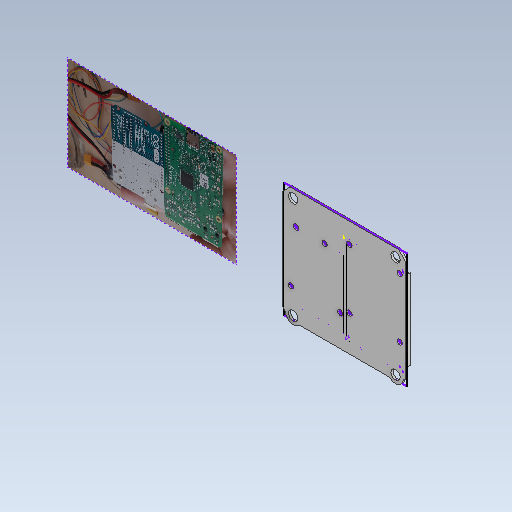
# Autodesk Inventor part: Крепление плат
Saved by Autodesk Inventor 2020 (Build 240168000, 168)
## iProperties
Created: 2021-04-20
Part Number: Крепление плат
Material: Типовые
Document SubType Name: Modeling
Designer: I_Love_U_Bogdan
Density: 1 g/cm^3
Appearance: По умолчанию
Author: I_Love_U_Bogdan
Autodesk Inventor part; units mm, degrees
ref_plane "YZ Plane" through (0, 0, 0) normal (1, 0, 0) x (0, 1, 0)
ref_plane "XZ Plane" through (0, 0, 0) normal (0, 1, 0) x (-1, 0, 0)
ref_plane "XY Plane" through (0, 0, 0) normal (0, 0, 1) x (1, 0, 0)
sketch "Эскиз2" plane through (0, 0, 0) normal (0, 0, 1) x (1, 0, 0)
  line L0 (-106.4716, 15.9838) -> (-106.4716, -76.8287) construction
  line L1 (-106.4716, -76.8287) -> (-271.4716, -76.8287) construction
  line L2 (-271.4716, -76.8287) -> (-271.4716, 15.9838) construction
  line L3 (-271.4716, 15.9838) -> (-106.4716, 15.9838) construction
  line L4 (4.5, 0) -> (54.5, 0)
  line L5 (57.5, -3) -> (57.5, -82)
  line L6 (54.5, -85) -> (4.5, -85)
  line L7 (1.5, -82) -> (1.5, -3)
  circle A0 centre (5, -3.5) radius 1.5
  circle A1 centre (54, -3.5) radius 1.5
  circle A2 centre (5, -61.5) radius 1.5
  circle A3 centre (54, -61.5) radius 1.5
  line L8 (-54.8, -14.8714) -> (-54.8, -80.9714)
  line L9 (-54.8, -80.9714) -> (-1.5, -80.9714)
  line L10 (-1.5, -80.9714) -> (-1.5, -14.8714)
  line L11 (-49.8, -11.8527) -> (-48.1279, -11.8527) construction
  circle A4 centre (-47.2, -14.8714) radius 1.5
  circle A5 centre (-19.3, -14.8714) radius 1.5
  circle A6 centre (-4.1, -65.6714) radius 1.5
  circle A7 centre (-52.3, -66.9714) radius 1.5
  line L12 (-16.4799, -14.8714) -> (-1.5, -14.8714)
  line L13 (-54.8, -14.8714) -> (-52.8, -14.8714)
  arc A8 (4.5, 0) -> (1.5, -3) centre (4.5, -3) ccw
  arc A9 (57.5, -3) -> (54.5, 0) centre (54.5, -3) ccw
  arc A10 (54.5, -85) -> (57.5, -82) centre (54.5, -82) ccw
  arc A11 (1.5, -82) -> (4.5, -85) centre (4.5, -82) ccw
  line L14 (-52.8, -14.8714) -> (-50.4525, -12.5239)
  line L15 (-52.8, -14.8714) -> (-49.4801, -14.8714) construction
  line L16 (-50.4525, -12.5239) -> (-18.8274, -12.5239)
  line L17 (-18.8274, -12.5239) -> (-16.4799, -14.8714)
  line L18 (4.5, -85.2) -> (54.5, -85.2)
  arc A12 (54.5, -85.2) -> (57.7, -82) centre (54.5, -82) ccw
  line L19 (57.7, -82) -> (57.7, -3)
  arc A13 (57.7, -3) -> (54.5, 0.2) centre (54.5, -3) ccw
  line L20 (54.5, 0.2) -> (4.5, 0.2)
  arc A14 (4.5, 0.2) -> (1.3, -3) centre (4.5, -3) ccw
  line L21 (1.3, -3) -> (1.3, -82)
  arc A15 (1.3, -82) -> (4.5, -85.2) centre (4.5, -82) ccw
  line L22 (-1.3, -81.1714) -> (-55, -81.1714)
  line L23 (-55, -81.1714) -> (-55, -14.6714)
  line L24 (-55, -14.6714) -> (-52.8828, -14.6714)
  line L25 (-52.8828, -14.6714) -> (-50.5353, -12.3239)
  line L26 (-50.5353, -12.3239) -> (-18.7446, -12.3239)
  line L27 (-18.7446, -12.3239) -> (-16.3971, -14.6714)
  line L28 (-16.3971, -14.6714) -> (-1.3, -14.6714)
  line L29 (-1.3, -14.6714) -> (-1.3, -81.1714)
  line L30 (-1.3, -81.1714) -> (1.3, -81.1714)
  line L31 (-1.3, -14.6714) -> (-1.3, -3.088)
  line L32 (-1.3, -3.088) -> (1.3012, -3.088)
  line L33 (4.5, -85.2) -> (54.5, -85.2)
  line L34 (54.5, -85.2) -> (54.5, -86.2)
  line L35 (54.5, -86.2) -> (4.5, -86.2)
  line L36 (4.5, -86.2) -> (4.5, -85.2)
  line L37 (57.7, -82) -> (58.7, -82)
  line L38 (58.7, -82) -> (58.7, -3.088)
  line L39 (58.7, -3.088) -> (57.7, -3.088)
  line L40 (57.7, -3.088) -> (57.7, -82)
  line L41 (-1.5, -81.1714) -> (-54.8, -81.1714)
  line L42 (-54.8, -81.1714) -> (-54.8, -82.1714)
  line L43 (-54.8, -82.1714) -> (-1.5, -82.1714)
  line L44 (-1.5, -82.1714) -> (-1.5, -81.1714)
  line L45 (-55, -80.9714) -> (-56, -80.9714)
  line L46 (-56, -80.9714) -> (-56, -14.8714)
  line L47 (-56, -14.8714) -> (-55, -14.8714)
  line L48 (-55, -14.8714) -> (-55, -80.9714)
  line L49 (-50.5353, -12.3239) -> (-18.7446, -12.3239)
  line L50 (-18.7446, -12.3239) -> (-18.7446, -11.3239)
  line L51 (-18.7446, -11.3239) -> (-50.5353, -11.3239)
  line L52 (-50.5353, -11.3239) -> (-50.5353, -12.3239)
  circle A16 centre (5, -61.5) radius 2.5
  circle A17 centre (54, -61.5) radius 2.5
  circle A18 centre (54, -3.5) radius 2.5
  circle A19 centre (5, -3.5) radius 2.5
  circle A20 centre (-19.3, -14.8714) radius 2.5
  circle A21 centre (-47.2, -14.8714) radius 2.5
  circle A22 centre (-4.1, -65.6714) radius 2.5
  circle A23 centre (-52.3, -66.9714) radius 2.5
  line L53 (4.5, 0.2) -> (54.5, 0.2)
  line L54 (54.5, 0.2) -> (54.5, 1.2)
  line L55 (54.5, 1.2) -> (4.5, 1.2)
  line L56 (4.5, 1.2) -> (4.5, 0.2)
  line L57 (-60, 16.2) -> (60, 16.2)
  line L58 (60, 16.2) -> (60, -96.2)
  line L59 (60, -96.2) -> (-60, -96.2)
  line L60 (-60, -96.2) -> (-60, 16.2)
  point P0 (0, 0)
  point P1 (57.5, -85)
  point P2 (57.5, 0)
  point P3 (1.5, -85)
  point P4 (1.3, -3.088)
  point P5 (-54.8, -81.1714)
  dimension "d159" = 9
  dimension "d40" = 56
  dimension "d41" = 85
  dimension "d42" = 1.5
  dimension "d43" = 3
  dimension "d44" = 3
  dimension "d45" = 49
  dimension "d46" = 3.5
  dimension "d47" = 3.5
  dimension "d48" = 3
  dimension "d49" = 3
  dimension "d50" = 49
  dimension "d51" = 3.5
  dimension "d52" = 58
  dimension "d55" = 165
  dimension "d60" = 53.3
  dimension "d70" = 3
  dimension "d71" = 3
  dimension "d74" = 0
  dimension "d76" = 3
  dimension "d77" = 3
  dimension "d78" = 15.3
  dimension "d79" = 14
  dimension "d82" = 27.9
  dimension "d83" = 2.5
  dimension "d84" = 5.1
  dimension "d85" = 15.2
  dimension "d86" = 50.8
  dimension "d90" = 3
  dimension "d92" = 50.8
  dimension "d93" = 50.8
  dimension "d98" = 45
  dimension "d99" = 135
  dimension "d101" = 2
  dimension "d104" = 2.3475
  dimension "d105" = 3.0187
  dimension "d106" = 10.5924
  dimension "d107" = 46.6279
  dimension "d108" = 48.3
  dimension "d113" = 1.5
  dimension "d114" = 0.2
  dimension "d115" = 0.2
  dimension "d118" = 1
  dimension "d119" = 1
  dimension "d120" = 1
  dimension "d121" = 1
  dimension "d122" = 1
  dimension "d123" = 1
  dimension "d124" = 1
  dimension "d125" = 1
  dimension "d126" = 1
  dimension "d127" = 1
  dimension "d128" = 1
  dimension "d129" = 1
  dimension "d130" = 1
  dimension "d131" = 1
  dimension "d133" = 10
  dimension "d134" = 15
  dimension "d135" = 60
  dimension "d136" = 120
  constraints: 114 end point, 24 centre point, 22 parallel, 18 point on circle, 14 horizontal, 12 perpendicular, 10 point on line, 8 tangent, 3 equal radius, 1 equal length, 1 vertical, 16 other
  measures "d40" distance of point (57.5, -85) point (1.5, -85)
  measures "d41" distance of point (57.5, 0) point (57.5, -85)
  measures "d42" distance from line of L7 point (0, 0)
  measures "d43" diameter of A0
  measures "d44" diameter of A1
  measures "d45" distance of A0.centre A1.centre
  measures "d46" distance from line of L7 A0.centre
  measures "d47" distance from line of L4 A0.centre
  measures "d48" diameter of A2
  measures "d49" diameter of A3
  measures "d50" distance of A3.centre A2.centre
  measures "d51" distance from line of L7 A2.centre
  measures "d52" distance of A0.centre A2.centre
  measures "d55" distance of L2.end L0.start
  measures "d60" distance of L9.end L8.end
  measures "d70" diameter of A5
  measures "d71" diameter of A4
  measures "d74" vertical distance of A5.centre A4.centre
  measures "d76" diameter of A6
  measures "d77" diameter of A7
  measures "d78" distance from line of A6.centre L9
  measures "d79" distance from line of L9 A7.centre
  measures "d82" distance of A4.centre A5.centre
  measures "d83" distance from line of L8 A7.centre
  measures "d84" horizontal distance of A4.centre A7.centre
  measures "d85" horizontal distance of A5.centre A6.centre
  measures "d86" vertical distance of A5.centre A6.centre
  measures "d90" radius of A8
  measures "d92" distance from line of L12 A6.centre
  measures "d93" distance from line of L13 A6.centre
  measures "d98" angle of L15 L14
  measures "d99" angle of L16 L17
  measures "d101" distance of L8.start L13.end
  measures "d104" distance between parallel lines of L16 L12
  measures "d105" distance between parallel lines of L12 L11
  measures "d106" distance from line of L10.end L17
  measures "d107" distance from line of L11.end L10
  measures "d108" distance from line of L11.start L10
  measures "d113" distance from line of point (0, 0) L10
  measures "d114" distance between parallel lines of L6 L18
  measures "d115" distance between parallel lines of L9 L22
  measures "d118" distance of L33.end L34.end
  measures "d119" distance of L39.end L38.end
  measures "d120" distance of L42.end L41.end
  measures "d121" distance of L46.end L47.end
  measures "d122" distance of L50.end L49.end
  measures "d123" radial gap between concentric circles of A2 A16
  measures "d124" radial gap between concentric circles of A3 A17
  measures "d125" radial gap between concentric circles of A1 A18
  measures "d126" radial gap between concentric circles of A0 A19
  measures "d127" radial gap between concentric circles of A4 A21
  measures "d128" radial gap between concentric circles of A7 A23
  measures "d129" radial gap between concentric circles of A6 A22
  measures "d130" radial gap between concentric circles of A20 A5
  measures "d131" distance of L54.end L53.end
  measures "d133" distance between parallel lines of L59 L35
  measures "d134" distance between parallel lines of L57 L55
  measures "d135" distance from line of point (0, 0) L58
  measures "d136" distance of L57.start L57.end
extrude "Выдавливание1" add sketch "Эскиз2" along normal blind 1 contours L4 A9 L5 A10 L6 A11 L7 A8 | A23 | L13 L14 L16 A21 A20 L17 L12 L10 L9 L8 | L8 L9 L10 L12 L17 A20 L27 L28 L29 L22 L23 L24 L25 L26 L16 A21 L14 L13 | A21 L16 | L16 A21 | A20 L27 L17 L16 | L16 L17 A20 | A20 L27 | L26 L52 L51 L50 | L31 L32 L21 L30 L29 | L44 L43 L42 L22 | L21 A14 L20 A13 L19 A12 L18 A15 | L23 L45 L46 L47 | L18 L34 L35 L36 | L56 L55 L54 L20 | L19 L39 L38 L37 | A16 | A17 | A18 | A19 | A22 | L57 L58 L59 L60
chamfer "Фаска1" distance 7 angle 45 4 edges at (-60, -96.2, 0.5) (60, -96.2, 0.5) (60, 16.2, 0.5) (-60, 16.2, 0.5)
extrude "Выдавливание2" add sketch "Эскиз2" against normal blind 3 contours A23 | A21 L16 | L16 A21 | A20 L27 L17 L16 | L16 L17 A20 | A20 L27 | A16 | A17 | A18 | A19 | A22
extrude "Выдавливание3" add sketch "Эскиз2" against normal blind 5 contours L26 L52 L51 L50 | L31 L32 L21 L30 L29 | L44 L43 L42 L22 | L23 L45 L46 L47 | L18 L34 L35 L36 | L56 L55 L54 L20 | L19 L39 L38 L37
fillet "Сопряжение1" radius 0.5 28 edges at (58.7, -82, -2.5) (57.7, -82, -2.5) (54.5, -86.2, -2.5) (54.5, -85.2, -2.5) (4.5, -86.2, -2.5) (4.5, -85.2, -2.5) (1.3, -81.1714, -2.5) (-1.3, -81.1714, -2.5) (-1.5, -82.1714, -2.5) (-1.5, -81.1714, -2.5) (-54.8, -82.1714, -2.5) (-54.8, -81.1714, -2.5) (-55, -80.9714, -2.5) (-56, -80.9714, -2.5) (-50.5353, -12.3239, -2.5) (-50.5353, -11.3239, -2.5) (-56, -14.8714, -2.5) (-55, -14.8714, -2.5) (-18.7446, -11.3239, -2.5) (-18.7446, -12.3239, -2.5) (-1.3, -3.088, -2.5) (1.3, -3.088, -2.5) (4.5, 0.2, -2.5) (4.5, 1.2, -2.5) (54.5, 0.2, -2.5) (54.5, 1.2, -2.5) (57.7, -3.088, -2.5) (58.7, -3.088, -2.5)
chamfer "Фаска2" distance 1 angle 45 8 edges at (52.5, -61.5, 1) (3.5, -61.5, 1) (-5.6, -65.6714, 1) (-53.8, -66.9714, 1) (-20.8, -14.8714, 1) (-48.7, -14.8714, 1) (3.5, -3.5, 1) (52.5, -3.5, 1)
sketch "Эскиз3" plane through (0, 0, 0) normal (0, 0, -1) x (-1, 0, 0)
  circle A0 centre (50, 8.2) radius 4.5
  line L0 (60, 9.2) -> (60, -89.2) projected
  line L1 (-53, 16.2) -> (53, 16.2) projected
  circle A1 centre (-50, 8.2) radius 4.5
  line L2 (-60, -89.2) -> (-60, 9.2) projected
  circle A2 centre (50, -91.2) radius 4.5
  line L3 (53, -96.2) -> (-53, -96.2) projected
  circle A3 centre (-50, -91.2) radius 4.5
  point P0 (0, 0)
  dimension "d150" = 9
  dimension "d151" = 10
  dimension "d152" = 8
  dimension "d153" = 9
  dimension "d154" = 8
  dimension "d155" = 10
  dimension "d156" = 9
  dimension "d157" = 5
  dimension "d158" = 10
  dimension "d159" = 9
  dimension "d160" = 10
  dimension "d161" = 5
  constraints: 4 centre point
  measures "d150" diameter of A0
  measures "d151" distance from line of L0 A0.centre
  measures "d152" distance from line of L1 A0.centre
  measures "d153" diameter of A1
  measures "d154" distance from line of L1 A1.centre
  measures "d155" distance from line of L2 A1.centre
  measures "d156" diameter of A2
  measures "d157" distance from line of L3 A2.centre
  measures "d158" distance from line of L0 A2.centre
  measures "d159" diameter of A3
  measures "d160" distance from line of L2 A3.centre
  measures "d161" distance from line of L3 A3.centre
extrude "Выдавливание4" cut sketch "Эскиз3" against normal blind 1
sketch "Эскиз4" plane through (0, 0, 0) normal (0, 0, -1) x (-1, 0, 0)
  circle A0 centre (50, -91.2) radius 4.5 projected
  circle A1 centre (-50, -91.2) radius 4.5 projected
  circle A2 centre (50, -91.2) radius 7.5
  circle A3 centre (-50, -91.2) radius 7.5
  point P0 (0, 0)
  dimension "d164" = 3
  dimension "d165" = 3
  constraints: 2 centre point
  measures "d164" radial gap between concentric circles of A0 A2
  measures "d165" radial gap between concentric circles of A1 A3
extrude "Выдавливание5" add sketch "Эскиз4" against normal blind 1
sketch "Эскиз5" plane through (0, 0, 0) normal (0, 0, -1) x (-1, 0, 0)
  line L0 (-54, -85.2) -> (-5, -85.2) projected
  arc A0 (-5, -86.2) -> (-5, -85.2) centre (-5, -85.7) ccw projected
  line L1 (-5, -86.2) -> (-54, -86.2) projected
  arc A1 (-54, -85.2) -> (-54, -86.2) centre (-54, -85.7) ccw projected
  circle A2 centre (-50, -91.2) radius 4.5 projected
  circle A3 centre (50, -91.2) radius 4.5 projected
  circle A4 centre (-5, -61.5) radius 2.5 projected
  circle A5 centre (4.1, -65.6714) radius 2.5 projected
  circle A6 centre (52.3, -66.9714) radius 2.5 projected
  circle A7 centre (-54, -61.5) radius 2.5 projected
  circle A8 centre (-5, -3.5) radius 2.5 projected
  circle A9 centre (19.3, -14.8714) radius 2.5 projected
  circle A10 centre (47.2, -14.8714) radius 2.5 projected
  circle A11 centre (-54, -3.5) radius 2.5 projected
  line L2 (54.3, -82.1714) -> (2, -82.1714) projected
  arc A12 (2, -81.1714) -> (2, -82.1714) centre (2, -81.6714) ccw projected
  line L3 (2, -81.1714) -> (54.3, -81.1714) projected
  arc A13 (54.3, -82.1714) -> (54.3, -81.1714) centre (54.3, -81.6714) ccw projected
  line L4 (-58.7, -81.5) -> (-58.7, -3.588) projected
  arc A14 (-57.7, -3.588) -> (-58.7, -3.588) centre (-58.2, -3.588) ccw projected
  line L5 (-57.7, -3.588) -> (-57.7, -81.5) projected
  arc A15 (-58.7, -81.5) -> (-57.7, -81.5) centre (-58.2, -81.5) ccw projected
  arc A16 (-5, 0.2) -> (-5, 1.2) centre (-5, 0.7) ccw projected
  line L6 (-5, 0.2) -> (-54, 0.2) projected
  arc A17 (-54, 1.2) -> (-54, 0.2) centre (-54, 0.7) ccw projected
  line L7 (-54, 1.2) -> (-5, 1.2) projected
  line L8 (56, -15.3714) -> (56, -80.4714) projected
  arc A18 (55, -80.4714) -> (56, -80.4714) centre (55.5, -80.4714) ccw projected
  line L9 (55, -80.4714) -> (55, -15.3714) projected
  arc A19 (56, -15.3714) -> (55, -15.3714) centre (55.5, -15.3714) ccw projected
  arc A20 (-57.4821, -91.7179) -> (-44.4098, -96.2) centre (-50, -91.2) ccw projected
  line L10 (44.4098, -96.2) -> (-44.4098, -96.2) projected
  arc A21 (44.4098, -96.2) -> (57.4821, -91.7179) centre (50, -91.2) ccw projected
  line L11 (60, -89.2) -> (57.4821, -91.7179) projected
  line L12 (60, 9.2) -> (60, -89.2) projected
  line L13 (53, 16.2) -> (60, 9.2) projected
  line L14 (-53, 16.2) -> (53, 16.2) projected
  line L15 (-60, 9.2) -> (-53, 16.2) projected
  line L16 (-60, -89.2) -> (-60, 9.2) projected
  line L17 (-57.4821, -91.7179) -> (-60, -89.2) projected
  line L18 (0.8, -81.1714) -> (-0.8, -81.1714) projected
  arc A22 (-1.3, -80.6714) -> (-0.8, -81.1714) centre (-0.8, -80.6714) ccw projected
  line L19 (-1.3, -80.6714) -> (-1.3, -3.588) projected
  arc A23 (-0.8, -3.088) -> (-1.3, -3.588) centre (-0.8, -3.588) ccw projected
  line L20 (-0.8, -3.088) -> (0.8, -3.088) projected
  arc A24 (1.3, -3.588) -> (0.8, -3.088) centre (0.8, -3.588) ccw projected
  line L21 (1.3, -3.588) -> (1.3, -80.6714) projected
  arc A25 (0.8, -81.1714) -> (1.3, -80.6714) centre (0.8, -80.6714) ccw projected
  arc A26 (50.0353, -12.3239) -> (50.0353, -11.3239) centre (50.0353, -11.8239) ccw projected
  line L22 (50.0353, -12.3239) -> (19.2446, -12.3239) projected
  arc A27 (19.2446, -11.3239) -> (19.2446, -12.3239) centre (19.2446, -11.8239) ccw projected
  line L23 (19.2446, -11.3239) -> (50.0353, -11.3239) projected
  circle A28 centre (50, 8.2) radius 4.5 projected
  circle A29 centre (-50, 8.2) radius 4.5 projected
  line L24 (52.5858, 15.2) -> (59, 8.7858)
  line L25 (59, 8.7858) -> (59, -88.7858)
  line L26 (59, -88.7858) -> (56.4994, -91.2864)
  arc A30 (44.8765, -95.2) -> (56.4994, -91.2864) centre (50, -91.2) ccw
  line L27 (44.8765, -95.2) -> (-44.8765, -95.2)
  arc A31 (-56.4994, -91.2864) -> (-44.8765, -95.2) centre (-50, -91.2) ccw
  line L28 (-56.4994, -91.2864) -> (-59, -88.7858)
  line L29 (-59, -88.7858) -> (-59, 8.7858)
  line L30 (-59, 8.7858) -> (-52.5858, 15.2)
  line L31 (-52.5858, 15.2) -> (52.5858, 15.2)
  line L32 (-59, -86.2864) -> (59, 3.7858) construction
  line L33 (-58.6966, -86.6838) -> (59.3034, 3.3883)
  line L34 (58.6966, 4.1832) -> (-59.3034, -85.8889)
  arc A32 (-59.3034, -85.8889) -> (-58.6966, -86.6838) centre (-59, -86.2864) ccw
  arc A33 (59.3034, 3.3883) -> (58.6966, 4.1832) centre (59, 3.7858) ccw
  line L35 (59, -86.2864) -> (-59, 3.7858) construction
  line L36 (59.3034, -85.8889) -> (-58.6966, 4.1832)
  line L37 (-59.3034, 3.3883) -> (58.6966, -86.6838)
  arc A34 (58.6966, -86.6838) -> (59.3034, -85.8889) centre (59, -86.2864) ccw
  arc A35 (-58.6966, 4.1832) -> (-59.3034, 3.3883) centre (-59, 3.7858) ccw
  circle A36 centre (-50, 8.2) radius 7.5
  circle A37 centre (50, 8.2) radius 7.5
  circle A38 centre (-50, -91.2) radius 7.5
  circle A39 centre (50, -91.2) radius 7.5
  point P0 (0, 0)
  point P1 (0, -41.2503)
  point P2 (0, -41.2503)
  point P3 (59, 4.2858)
  point P4 (0, -40.6213)
  point P5 (-59, 4.2858)
  point P6 (-59, 3.1568)
  point P7 (-0.8241, -41.2503)
  point P8 (-59, -85.6573)
  point P9 (-59, -86.7864)
  point P10 (0, -41.8793)
  point P11 (59, -86.7864)
  point P12 (59, -85.6573)
  point P13 (0.8241, -41.2503)
  point P14 (59, 3.1568)
  point P15 (57.45, -90.3357)
  point P16 (43.6557, -95.2)
  point P17 (-43.6557, -95.2)
  point P18 (-44.4098, -86.2)
  point P19 (-45.5, -85.2)
  point P20 (-57.45, -90.3357)
  point P21 (-47.3074, 15.2)
  point P22 (-57.063, 10.7228)
  point P23 (-52.6926, 1.2)
  point P24 (-47.3074, 1.2)
  point P25 (47.3074, 15.2)
  point P26 (57.063, 10.7228)
  dimension "d105" = 3.0187
  dimension "d168" = 1
  dimension "d171" = 1
  dimension "d172" = 1
  dimension "d173" = 5
  dimension "d174" = 5
  dimension "d175" = 5
  dimension "d176" = 5
  dimension "d177" = 3
  dimension "d178" = 3
  dimension "d179" = 3
  dimension "d180" = 3
  constraints: 32 end point, 12 point on circle, 10 centre point, 8 tangent, 4 point on line, 2 midpoint, 2 parallel, 9 other
  measures "d168" distance between parallel lines of L14 L31
  measures "d171" diameter of A33
  measures "d172" diameter of A35
  measures "d173" distance of L29.end L35.end
  measures "d174" distance of L24.end L32.end
  measures "d175" vertical distance of L28.start L32.start
  measures "d176" vertical distance of L35.start L26.end
  measures "d177" radial gap between concentric circles of A29 A36
  measures "d178" radial gap between concentric circles of A28 A37
  measures "d179" radial gap between concentric circles of A2 A38
  measures "d180" radial gap between concentric circles of A3 A39
extrude "Выдавливание6" add sketch "Эскиз5" along normal blind 1 contours A1 L1 A38 L27 A31 L28 L0 | A38 L17 L16 L15 L14 L13 L12 L11 A39 L26 L25 A34 L36 L33 A33 L24 A37 L31 A36 L30 L29 A35 L37 L34 A32 L28 | L28 A31 L27 A38 A20 | L27 A39 L10 A38 | A32 L34 L29 | L29 L34 L19 L33 A32 | A39 L26 A30 L27 | L27 A30 L26 A39 A21 | L37 A35 L29 | L29 A35 L36 A17 L6 L19 L37 A11 | L34 L37 L33 L19 | A11 L37 | L19 L36 L34 L37 | L34 L36 L33 L37 | L33 L36 L21 L37 | A34 L37 L2 A13 L36 L25 | L25 L36 A34 | L34 L21 L33 L36 | L21 L36 L3 L37 | A36 L31 L30 | L30 L31 A36 L7 | L36 L6 A17 | L34 L22 L33 L21 | L3 L36 A13 L2 L37 | L33 L23 L34 A33 L25 | L25 A33 L33 | L34 L23 L33 L22 | A37 L24 L31 | L31 L24 A37 picked at (-52.4477, -1.7689)
